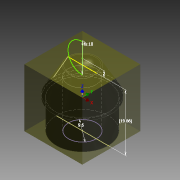
# Autodesk Inventor part: Rod End 20mm Formula-driven
Saved by Autodesk Inventor 2,015 SP1 (Build 190203100, 203)
## iProperties
Created: 2015-04-29
Part Number: Rod End 20mm Formula-driven
Material: Generic
Document SubType Name: Modeling
Designer: tsmember
Density: 1 g/cm^3
Appearance: Default
Mass: 3.13491 g
Surface Area: 20.0477 cm^2
Volume: 3.13491 cm^3
Author: tsmember
Autodesk Inventor part; units mm, degrees
ref_plane "YZ Plane" through (0, 0, 0) normal (1, 0, 0) x (0, 1, 0)
ref_plane "XZ Plane" through (0, 0, 0) normal (0, 1, 0) x (-1, 0, 0)
ref_plane "XY Plane" through (0, 0, 0) normal (0, 0, 1) x (1, 0, 0)
sketch "RingSketch" plane through (0, 0, 0) normal (0, 0, 1) x (1, 0, 0)
  circle A0 centre (0, 0) radius 10
  dimension "RingDia" = 20
  constraints: 1 centre point, 1 coincident
  measures "RingDia" diameter of A0
extrude "Ring" add sketch "RingSketch" against normal blind 1
sketch "ShankSketch" plane through (0, 0, -1) normal (0, 0, -1) x (-1, 0, 0)
  circle A0 centre (0, 0) radius 8.975
  dimension "ShankDia" = 17.95
  constraints: 1 centre point, 1 coincident
  measures "ShankDia" diameter of A0
extrude "Shank" add sketch "ShankSketch" along normal blind 10
sketch "ConeSketch" plane through (0, 0, 0) normal (1, 0, 0) x (0, 1, 0)
  line L0 (0, 0) -> (10, 0)
  line L1 (10, 0) -> (5, 8.6603)
  line L2 (5, 8.6603) -> (0, 8.6603)
  line L3 (0, 8.6603) -> (0, 0)
  line L4 (-10, 0) -> (10, 0) projected
  dimension "ConeAngle" = 60
  dimension "ConeBase" = 10
  dimension "ConeTipDia" = 5
  constraints: 8 end point, 1 horizontal, 1 parallel, 1 perpendicular
  measures "ConeAngle" angle of L0 L1
  measures "ConeBase" distance of L0.start L0.end
  measures "ConeTipDia" distance of L1.end L2.end
revolve "Cone" add sketch "ConeSketch" angle 360 about axis through (0, 0, 8.6603) along (0, 0, -1)
sketch "SocketSketch" plane through (0, 0, 0) normal (0, 1, 0) x (-1, 0, 0)
  arc A0 (0, 5.6603) -> (0, 15.6603) centre (0, 10.6603) ccw
  line L0 (0, 15.6603) -> (0, 5.6603)
  line L1 (-5, 8.6603) -> (5, 8.6603) projected
  line L2 (5, 8.6603) -> (10, 0) projected
  point P0 (0, 0)
  dimension "RecessDia" = 10
  dimension "BallOffset" = 2
  constraints: 2 end point, 2 point on circle, 1 centre point, 1 vertical
  measures "RecessDia" diameter of A0
  measures "BallOffset" distance from line of L1 A0.centre
revolve "Socket" cut sketch "SocketSketch" angle 360 about axis through (0, 0, 15.6603) along (0, 0, -1)
sketch "MagnetHoleSketch" plane through (0, 0, -11) normal (0, 0, -1) x (-1, 0, 0)
  circle A0 centre (0, 0) radius 4.8
  dimension "MagnetHoleDia" = 9.6
  constraints: 1 centre point, 1 coincident
  measures "MagnetHoleDia" diameter of A0
extrude "MagnetHole" cut sketch "MagnetHoleSketch" against normal blind 16.1603
sketch "PartLength" plane through (0, 0, 0) normal (0, 1, 0) x (-1, 0, 0)
  line L0 (-5, 8.6603) -> (5, 8.6603) projected
  line L1 (-8.975, -11) -> (8.975, -11) projected
  point P0 (0, 0)
  dimension "PartLen" = 19.6603
  measures "PartLen" distance between parallel lines of L1 L0
equation "\"ConeBase\" = 0.5 * RingDia"
equation "\"ConeTipDia\" = 0.5 * BallDia"
equation "\"RecessDia\" = BallDia"
equation "\"BallDia\" = 10"
